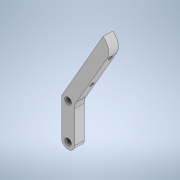
# Autodesk Inventor part: Gripper 5-2
Saved by Autodesk Inventor 2021 (Build 250183000, 183)
## iProperties
Created: 2022-01-08
Part Number: Gripper 5-2
Material: Generic
Document SubType Name: Modeling
Designer: Łukasz
Density: 1 g/cm^3
Appearance: Default
Author: Łukasz
Autodesk Inventor part; units mm, degrees
ref_plane "YZ Plane" through (0, 0, 0) normal (1, 0, 0) x (0, 1, 0)
ref_plane "XZ Plane" through (0, 0, 0) normal (0, 1, 0) x (-1, 0, 0)
ref_plane "XY Plane" through (0, 0, 0) normal (0, 0, 1) x (1, 0, 0)
sketch "Sketch1" plane through (0, 0, 0) normal (0, 0, 1) x (1, 0, 0)
  circle A0 centre (0, 0) radius 2
  arc A1 (-4, 0) -> (4, 0) centre (0, 0) ccw
  line L0 (0, 0) -> (0, 22) construction
  circle A2 centre (0, 22) radius 2
  arc A3 (-3.7993, 23.2511) -> (-4, 22) centre (0, 22) ccw
  line L1 (0, 22) -> (25, 65.3013) construction
  circle A4 centre (25, 65.3013) radius 2
  arc A5 (27, 61.8372) -> (21.2007, 66.5524) centre (25, 65.3013) ccw
  line L2 (-4, 0) -> (-4, 22)
  line L3 (4, 0) -> (4, 22)
  line L4 (-3.7993, 23.2511) -> (17.6088, 60.331)
  line L5 (24, 56.641) -> (4, 22)
  line L6 (30.6468, 62.0411) -> (28.537, 63.2592)
  line L7 (27, 61.8372) -> (28, 63.5692)
  line L8 (21.2007, 66.5524) -> (17.6088, 60.331)
  line L9 (21.0718, 67.5692) -> (19.4047, 68.5317)
  line L10 (21.2007, 66.5524) -> (21.6088, 67.2592)
  arc A6 (24, 56.641) -> (21.0718, 67.5692) centre (17.0718, 60.641) ccw
  line L11 (27, 61.8372) -> (24, 56.641)
  point P0 (21.5269, 67.2857)
  point P1 (21.5967, 67.2384)
  dimension "d0" = 4
  dimension "d1" = 8
  dimension "d2" = 22
  dimension "d3" = 4
  dimension "d4" = 8
  dimension "d5" = 50
  dimension "d6" = 150
  dimension "d7" = 4
  dimension "d8" = 8
  dimension "d13" = 8
  constraints: 24 end point, 8 point on circle, 7 centre point, 6 coincident, 5 point on line, 4 tangent, 2 parallel, 2 perpendicular, 1 vertical
  measures "d0" diameter of A0
  measures "d1" diameter of A1
  measures "d2" distance of L0.start L0.end
  measures "d3" diameter of A2
  measures "d4" diameter of A3
  measures "d5" distance of L1.start L1.end
  measures "d6" angle of L0 L1
  measures "d7" diameter of A4
  measures "d8" diameter of A5
  measures "d13" radius of A6
extrude "Extrusion1" add sketch "Sketch1" along normal blind 6 contours L2 A3 L4 L8 L10 A6 A4 L5 L3 A1 | A4 A6 picked at (23.7732, 64.4877)
fillet "Fillet1" radius 8 1 edges at (4, 22, 3)
sketch "Sketch2" plane through (-3.7993, 23.2511, 0) normal (-0.866, 0.5, 0) x (0, 0, 1)
  line L0 (0, 42.8162) -> (6, 42.8162) projected
  circle A0 centre (3, 17.7921) radius 1.25
  circle A1 centre (3, 40.7921) radius 1.25
  line L1 (0, 50.7921) -> (6, 50.7921) projected
  line L2 (0, 0) -> (6, 0) projected
  line L3 (-2.4062, 7.7921) -> (9.3174, 7.7921)
  point P0 (0, -18.2364)
  dimension "d15" = 2.5
  dimension "d16" = 2.5
  dimension "d17" = 10
  dimension "d19" = 43
  dimension "d20" = 10
  constraints: 2 centre point, 2 end point, 1 horizontal
  measures "d15" diameter of A0
  measures "d16" diameter of A1
  measures "d17" distance from line of L1 A1.centre
  measures "d19" distance between parallel lines of L1 L3
  measures "d20" distance from line of L3 A0.centre
extrude "Extrusion2" cut sketch "Sketch2" against normal blind 10
body "Solid1"
